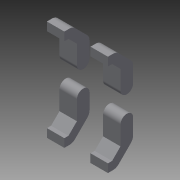
# Autodesk Inventor part: Bastion Feet
Saved by Autodesk Inventor 2014 SP1 (Build 180222100, 222)
## iProperties
Created: 2016-12-20
Part Number: Bastion Feet
Material: Generic
Document SubType Name: Modeling
Designer: potato
Density: 1 g/cm^3
Appearance: Default
Author: potato
Autodesk Inventor part; units mm, degrees
ref_plane "YZ Plane" through (0, 0, 0) normal (1, 0, 0) x (0, 1, 0)
ref_plane "XZ Plane" through (0, 0, 0) normal (0, 1, 0) x (-1, 0, 0)
ref_plane "XY Plane" through (0, 0, 0) normal (0, 0, 1) x (1, 0, 0)
sketch "Sketch1" plane through (0, 0, 0) normal (1, 0, 0) x (0, 1, 0)
  line L0 (330, 82.5) -> (330, 48.569)
  line L1 (-330, 48.569) -> (-330, 82.5)
  line L2 (96.2496, -82.5) -> (198.931, -82.5)
  line L3 (234.852, -67.621) -> (315.121, 12.648)
  line L4 (330, 82.5) -> (275.0088, 82.5)
  line L5 (275.0088, 82.5) -> (275.0088, 55.036)
  line L6 (96.2494, 0) -> (219.9728, 0)
  line L7 (219.9728, 0) -> (275.0088, 55.036)
  line L8 (-234.852, -67.621) -> (-315.121, 12.648)
  line L9 (-275.009, 82.5) -> (-275.009, 55.036)
  line L10 (-96.2496, 0) -> (-219.973, 0)
  line L11 (-219.973, 0) -> (-275.009, 55.036)
  line L12 (-330, 82.5) -> (-275.009, 82.5)
  line L13 (275.0088, 82.5) -> (330, 82.5)
  line L14 (198.931, -82.5) -> (96.25, -82.5)
  line L15 (-96.2496, -82.5) -> (-198.931, -82.5)
  arc A0 (-96.2496, -82.5) -> (-96.2496, 0) centre (-96.25, -41.25) ccw
  arc A1 (96.2494, 0) -> (96.2496, -82.5) centre (96.2498, -41.25) ccw
  arc A2 (-234.852, -67.621) -> (-198.931, -82.5) centre (-198.931, -31.7) ccw
  arc A3 (-330, 48.569) -> (-315.121, 12.648) centre (-279.2, 48.569) ccw
  arc A4 (198.931, -82.5) -> (234.852, -67.621) centre (198.931, -31.7) ccw
  arc A5 (315.121, 12.648) -> (330, 48.569) centre (279.2, 48.569) ccw
  point P0 (219.973, -82.5)
  point P1 (-219.973, -82.5)
  point P2 (330, 27.527)
  point P3 (-330, 27.527)
  constraints: 32 end point, 13 point on circle, 9 point on line, 8 tangent, 6 centre point, 5 parallel, 4 perpendicular, 2 equal radius, 2 horizontal
extrude "Extrusion1" add sketch "Sketch1" along normal mid plane 400
sketch "Sketch6" plane through (-200, 275.0088, 82.5) normal (0, 0, 1) x (1, 0, 0)
  line L0 (0, 0) -> (400, 0) projected
  line L1 (400, 54.9912) -> (0, 54.9912) projected
  line L2 (0, 0) -> (114.3, 0)
  line L3 (400, 54.9912) -> (285.7, 54.9912)
  line L4 (114.3, 0) -> (285.7, 0)
  line L5 (285.7, 0) -> (285.7, 54.9912)
  line L6 (285.7, 54.9912) -> (114.3, 54.9912)
  line L7 (114.3, 54.9912) -> (114.3, 0)
  line L8 (0, -605.6334) -> (114.3, -605.6334)
  line L9 (114.3, -605.6334) -> (285.7, -605.6334)
  line L10 (285.7, -605.6334) -> (285.7, 54.9912)
  line L11 (285.7, 54.9912) -> (114.3, 54.9912)
  line L12 (114.3, 54.9912) -> (114.3, -605.6334)
  point P0 (200, -275.0088)
  dimension "d39" = 114.3
  dimension "d40" = 114.3
  dimension "d41" = 114.3
  constraints: 22 end point, 4 parallel, 3 perpendicular, 2 horizontal, 2 point on line
  measures "d39" distance of L0.start L2.end
  measures "d40" distance of L1.start L3.end
  measures "d41" distance of L8.start L8.end
extrude "Extrusion6" cut sketch "Sketch6" against normal blind 165
body "Solid1"
